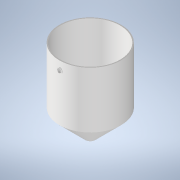
# Autodesk Inventor part: swirl filter
Saved by Autodesk Inventor 2020 (Build 240168000, 168)
## iProperties
Created: 2019-09-24
Part Number: swirl filter
Material: Generic
Document SubType Name: Modeling
Designer: a.komeijani
Density: 1 g/cm^3
Appearance: Default
Author: a.komeijani
Autodesk Inventor part; units mm, degrees
ref_plane "YZ Plane" through (0, 0, 0) normal (1, 0, 0) x (0, 1, 0)
ref_plane "XZ Plane" through (0, 0, 0) normal (0, 1, 0) x (-1, 0, 0)
sketch "Sketch1" plane through (0, 0, 0) normal (0, 0, 1) x (1, 0, 0)
  line L0 (542.1294, 0) -> (542.1294, -1000)
  line L1 (542.1294, -1000) -> (82.51, -1459.6194)
  line L2 (-7.8706, -896.0873) -> (-7.8706, -498.6597)
  line L3 (542.1294, 0) -> (542.1294, 0)
  line L4 (82.51, -1459.6194) -> (32.51, -1459.6194)
  line L5 (32.51, -1459.6194) -> (32.51, -1439.6194)
  line L6 (32.51, -1439.6194) -> (82.51, -1439.6194)
  line L7 (82.51, -1439.6194) -> (522.1294, -1000)
  line L8 (522.1294, -1000) -> (522.1294, 0)
  line L9 (522.1294, 0) -> (542.1294, 0)
  point P0 (0, 0)
  dimension "d0" = 1000
  dimension "d1" = 650
  dimension "d2" = 0
  dimension "d3" = 135
  dimension "d4" = 550
  dimension "d29" = 0
  dimension "d30" = 0
  dimension "d31" = 50
  dimension "d41" = 20
  constraints: 20 end point, 4 vertical, 2 horizontal, 2 parallel, 2 perpendicular, 1 coincident, 2 other
  measures "d0" distance of L0.start L0.end
  measures "d1" distance of L0.end L1.end
  measures "d2" distance of L1.end L4.start
  measures "d3" angle of L1 L0
  measures "d4" distance between parallel lines of L0 L2
  measures "d29" distance from line of point (0, 0) L3
  measures "d30" distance of L0.start L3.end
  measures "d31" distance of L4.start L4.end
  measures "d41" distance of L4.end L5.end
ref_plane "Work Plane6" through (-566.8771, -58.4878, 0) normal (0, -1, 0) x (1, 0, 0)
revolve "Revolution1" add sketch "Sketch1" angle 360 about axis through (-7.8706, -896.0873, 0) along (0, 1, 0)
ref_plane "Work Plane10" through (-7.8706, -500, 550) normal (0, 0, 1) x (1, 0, 0)
sketch "Sketch31" plane through (-7.8706, -500, 550) normal (0, 0, 1) x (1, 0, 0)
  circle A0 centre (7.8706, 350) radius 50
  circle A1 centre (7.8706, 350) radius 40
  line L0 (-550, 500) -> (550, 500) projected
  line L1 (7.8706, -1251.5433) -> (7.8706, 791.9239) projected
  point P0 (7.8706, 500)
  dimension "d102" = 100
  dimension "d103" = 80
  dimension "d104" = 150
  dimension "d105" = 0
  constraints: 2 centre point, 1 concentric
  measures "d102" diameter of A0
  measures "d103" diameter of A1
  measures "d104" distance from line of L0 A0.centre
  measures "d105" distance from line of L1 A0.centre
extrude "Extrusion15" add sketch "Sketch31" along normal blind 10 contours A0 L1 A1 | L1 A1 A0
sketch "Sketch32" plane through (-7.8706, -500, 550) normal (0, 0, 1) x (1, 0, 0)
  circle A0 centre (7.8706, 350) radius 40
  circle A1 centre (7.8706, 350) radius 40 projected
  point P0 (7.8706, 500)
  dimension "d108" = 80
  constraints: 1 centre point, 1 concentric
  measures "d108" diameter of A0
extrude "Extrusion16" cut sketch "Sketch32" against normal blind 50
body "Solid3"
